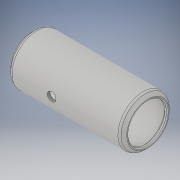
# Autodesk Inventor part: 007-0.79752
Saved by Autodesk Inventor 2018 (Build 220112000, 112)
## iProperties
Created: 2019-01-16
Part Number: 007-0.79752
Material: Generic
Catalog Web Link: www.cadenas.de
Description: Tube-Original Line - Standard Air Cylinders
Vendor: BIMBA
Document SubType Name: Modeling
Designer: s-4008082
Manufacturer: BIMBA
Mass: 0.278317 g
Surface Area: 11.7617 cm^2
Volume: 0.278317 cm^3
Density: 1 g/cm^3
Appearance: PSOLRGB-180-180-180
Category: PARTsolutions
Company: BIMBA
Title: 007-0.79752
Author: Cadenas PARTsolutions
Comments: Original Line - Standard Air Cylinders
PSOL_IDENT_0: {$CADENAS_DATA\23d-libs\bimba\bimba\bimba_imperial\bimba_full_line\original_line_cylinders\standard_
PSOL_IDENT_1: air_cylinders\tube.prj},199 {VTYP=3D},{NB=007-0.79752},{LINA=007-0.79752},{NN=Tube},{DATE=21.03.2018
PSOL_IDENT_2: 14:31:21},{GEOMDATE=18.02.2011 00:00:00},{VERSION=},{LINEID=10},{WBVAR=MNT,ACTING,NR,L,FOURHOLES,SR
PSOL_IDENT_3: },{WBNUMERIC=L,FOURHOLES}  {NB=007-0.79752},{LINA=007-0.79752},{KT=DUMMY},{PN=007-0.79752},{BORE=0.3
PSOL_IDENT_4: 1250000},{BOREPN=007},{MNT=},{MNTALG='' , 'Front Nose' , 'BF' , 'Front Block'},{ACTING=},{ACTINGALG=
PSOL_IDENT_5: '' , 'Single Acting' , 'R' , 'Reverse/Double Acting' },{NR=},{NRALG= '' , 'Without Non-rotating Rod'
PSOL_IDENT_6: , 'NR' , 'With Non-rotating Rod' },{L=0.7975},{OD=0.3590},{ODN=0.3590},{ODP=0.6050},{ODB=0.0000},{I
PSOL_IDENT_7: D=0.3215},{DV=0.09400000},{LV=0.37500000},{LV1=0.03000000},{G=0.0220},{FOURHOLES=2},{AA=0.3250},{BB=
PSOL_IDENT_8: 0.0620},{SR=},{SRALG= 'C' , 'Carbon Steel Rod' , 'SR' , '303 Stainless Steel Rod' , '' , '303 Stainl
PSOL_IDENT_9: ess Steel Rod'}
NN: Tube
NT: Original Line - Standard Air Cylinders
NB: 007-0.79752
NBSYN: $PN.
LINA: 007-0.79752
BORE: 0
BOREPN: 007
MNT: Front Nose
MNTALG: '' , 'Front Nose' , 'BF' , 'Front Block'
ACTING: Single Acting
NR: Without Non-rotating Rod
L: 0.7975
ODN: 0.359
ODP: 0.605
ODB: 0
ID: 0.3215
DV: 0.094
LV: 0.375
LV1: 0.03
G: 0.022
FOURHOLES: 2
AA: 0.325
BB: 0.062
SR: 303 Stainless Steel Rod
SUPPLIER: BIMBA
ARTICLENO: 007-0.79752
BOMINFO: 007-0.79752
CREATOR: CADENAS GmbH
Autodesk Inventor part; units mm, degrees
sketch "Sketch_1" plane through (0, 0, 0) normal (0, 0, 1) x (1, 0, 0)
  line L0 (20.2565, 0) -> (0, 0)
  arc A0 (-0.445, 3.8695) -> (-0.445, 3.6899) centre (-0.3552, 3.7797) ccw
  line L1 (-0.445, 3.6899) -> (-0.2794, 3.5242)
  line L2 (-0.2794, 3.5242) -> (0, 3.5242)
  line L3 (0, 3.5242) -> (0.5588, 4.0831)
  line L4 (0.5588, 4.0831) -> (19.6977, 4.0831)
  line L5 (19.6977, 4.0831) -> (20.2565, 3.5242)
  line L6 (20.2565, 3.5242) -> (20.5359, 3.5242)
  line L7 (20.5359, 3.5242) -> (20.7015, 3.6899)
  arc A1 (20.7015, 3.6899) -> (20.7015, 3.8695) centre (20.6117, 3.7797) ccw
  line L8 (20.7015, 3.8695) -> (20.1754, 4.3956)
  arc A2 (20.1754, 4.3956) -> (19.7802, 4.5593) centre (19.7803, 4.0005) ccw
  line L9 (19.7802, 4.5593) -> (0.4763, 4.5593)
  arc A3 (0.4763, 4.5593) -> (0.0811, 4.3956) centre (0.4762, 4.0005) ccw
  line L10 (0.0811, 4.3956) -> (-0.445, 3.8695)
  constraints: 22 end point, 8 point on circle, 4 centre point
revolve "Revolution1" add sketch "Sketch_1" angle 360 about axis through (20.2565, 0, 0) along (1, 0, 0)
sketch "Sketch_4" plane through (0, 0, 0) normal (0, 0, 1) x (1, 0, 0)
  circle A0 centre (7.6962, 0) radius 0.7874
  constraints: 1 centre point
extrude "Extrusion1" cut sketch "Sketch_4" along normal blind 4.5593
ref_plane "cp1_XY" through (10.1283, 4.5593, 0) normal (1, 0, 0) x (0, 0, -1)
ref_plane "cp1_YZ" through (10.1283, 4.5593, 0) normal (0, 0, -1) x (0, 1, 0)
ref_plane "cp1_ZX" through (10.1283, 4.5593, 0) normal (0, 1, 0) x (1, 0, 0)
ref_plane "cp2_XY" through (10.1283, 0, -4.5593) normal (1, 0, 0) x (0, 0, -1)
ref_plane "cp2_YZ" through (10.1283, 0, -4.5593) normal (0, 0, -1) x (0, 1, 0)
ref_plane "cp2_ZX" through (10.1283, 0, -4.5593) normal (0, 1, 0) x (1, 0, 0)
ref_plane "cp3_XY" through (10.1283, -4.5593, 0) normal (1, 0, 0) x (0, 0, -1)
ref_plane "cp3_YZ" through (10.1283, -4.5593, 0) normal (0, 0, -1) x (0, 1, 0)
ref_plane "cp3_ZX" through (10.1283, -4.5593, 0) normal (0, 1, 0) x (1, 0, 0)
ref_plane "cp4_XY" through (10.1283, 0, 4.5593) normal (1, 0, 0) x (0, 0, -1)
ref_plane "cp4_YZ" through (10.1283, 0, 4.5593) normal (0, 0, -1) x (0, 1, 0)
ref_plane "cp4_ZX" through (10.1283, 0, 4.5593) normal (0, 1, 0) x (1, 0, 0)
ref_plane "tube_front_XY" through (0, 0, 0) normal (1, 0, 0) x (0, 0, -1)
ref_plane "tube_front_YZ" through (0, 0, 0) normal (0, 0, -1) x (0, 1, 0)
ref_plane "tube_front_ZX" through (0, 0, 0) normal (0, 1, 0) x (1, 0, 0)
ref_plane "tube_rear_XY" through (20.2565, 0, 0) normal (1, 0, 0) x (0, 0, -1)
ref_plane "tube_rear_YZ" through (20.2565, 0, 0) normal (0, 0, -1) x (0, 1, 0)
ref_plane "tube_rear_ZX" through (20.2565, 0, 0) normal (0, 1, 0) x (1, 0, 0)
body "Solid1"
